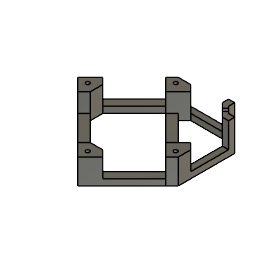
台2 v5 (Autodesk Fusion 360 design; units mm, degrees)
Autodesk Fusion 360 part; units mm, degrees
sketch "スケッチ1" plane through (0, 0, 0) normal (0, 0, 1) x (1, 0, 0)
  line L0 (0, 0) -> (-55, 0)
  line L1 (0, 0) -> (0, -5)
  line L2 (-10, -5) -> (-50, -5)
  line L3 (0, 0) -> (0, -55)
  line L4 (-5, -50) -> (-5, -10)
  line L5 (-5, -10) -> (-10, -5)
  line L6 (-5, -50) -> (-50, -5)
  line L7 (-5, -60) -> (-60, -5)
  line L8 (-60, -5) -> (-55, 0)
  line L9 (0, -55) -> (-5, -60)
  constraint coincident L0.start L1.start
  constraint horizontal L0
  constraint perpendicular L0 L1
  constraint perpendicular L1 L2
  constraint perpendicular L0 L3
  constraint perpendicular L2 L4
  constraint parallel L6 L7
  constraint perpendicular L6 L8
  constraint perpendicular L7 L9
extrude "押し出し1" add sketch "スケッチ1" along normal blind 5
sketch "スケッチ2" plane through (0, 0, 0) normal (0, 0, 1) x (1, 0, 0)
  line L0 (0, 0, 5) -> (-55, 0, 5)
  line L1 (-10, -5, 5) -> (-10, 0, 5)
  line L2 (-10, -5, 5) -> (-5, -10, 5)
  line L3 (0, -55, 5) -> (0, 0, 5)
  line L4 (-5, -10, 5) -> (0, -10, 5)
  line L5 (-60, -5, 5) -> (-5, -60, 5)
  line L6 (-5, -60, 5) -> (0, -55, 5)
  line L7 (-55, 0, 5) -> (-60, -5, 5)
  line L8 (-10, -55, 5) -> (-15, -50, 5)
  line L9 (-5, -10, 5) -> (-5, -50, 5)
  line L10 (0, -45, 5) -> (-5, -40, 5)
  line L11 (-15, -50, 5) -> (-5, -40, 5)
  line L12 (-50, -5, 5) -> (-10, -5, 5)
  line L13 (-50, -15, 5) -> (-40, -5, 5)
  line L14 (-45, 0, 5) -> (-40, -5, 5)
  line L15 (-55, -10, 5) -> (-50, -15, 5)
  point P0 (-10, -5)
  point P1 (-10, -5)
  point P2 (-5, -10)
  point P3 (-5, -50)
  point P4 (-50, -5)
  constraint coincident P0 P1
  constraint coincident P1 P0
extrude "押し出し2" add sketch "スケッチ2" along normal blind 50 contours L0 L1 L2 L3 L4 | L0 L5 L7 L13 L14 L15 | L3 L5 L6 L8 L10 L11 in plane through (0, 0, 5) normal (0, 0, 1)
sketch "スケッチ3" plane through (0, 0, 0) normal (0, 0, 1) x (1, 0, 0)
extrude "押し出し3" cut 2 faces at (-50, -5, 55) (-5, -50, 55) along direction (0, 0, -1) blind 30
sketch "スケッチ4" plane through (0, 0, 0) normal (0, 0, 1) x (1, 0, 0)
  line L0 (-60, -5) -> (-95, -40)
  line L1 (-95, -40) -> (-40, -95)
  line L2 (-40, -95) -> (-5, -60)
  line L3 (-5, -60) -> (-60, -5)
  line L4 (-55, -10) -> (-80, -35)
  line L5 (-80, -45) -> (-45, -80)
  line L6 (-35, -80) -> (-10, -55)
  line L7 (-35, -80) -> (-45, -80)
  line L8 (-80, -35) -> (-80, -45)
  point P0 (-5, -60)
  constraint perpendicular L0 L1
  constraint coincident P0 L2.end
  constraint coincident L3 L4.start
  constraint perpendicular L3 L4
  constraint perpendicular L4 L5
  constraint coincident L3 L6.end
  constraint perpendicular L3 L6
  constraint horizontal L7
  constraint perpendicular L7 L8
extrude "押し出し4" add sketch "スケッチ4" along normal blind 5 contours L0 L1 L2 L3 L4 L5 L6 L7 L8
sketch "スケッチ5" plane through (0, 0, 5) normal (0, 0, 1) x (-1, 0, 0)
  line L0 (55, 10) -> (60, 5)
  line L1 (60, 5) -> (95, 40)
  line L2 (95, 40) -> (40, 95)
  line L3 (40, 95) -> (5, 60)
  line L4 (10, 55) -> (35, 80)
  line L5 (35, 80) -> (45, 80)
  line L6 (45, 80) -> (80, 45)
  line L7 (80, 45) -> (80, 35)
  line L8 (80, 35) -> (55, 10)
  line L9 (80, 35) -> (85, 30)
  line L10 (80, 45) -> (85, 50)
  line L11 (45, 80) -> (50, 85)
  line L12 (35, 80) -> (30, 85)
  line L13 (5, 60) -> (10, 55)
  constraint coincident L7.end L8.start
  constraint coincident L1 L9.end
  constraint perpendicular L1 L9
  constraint coincident L6.end L7.start
  constraint coincident L2 L10.end
  constraint perpendicular L2 L10
  constraint coincident L5.end L6.start
  constraint coincident L2 L11.end
  constraint perpendicular L2 L11
  constraint coincident L4.end L5.start
  constraint coincident L3 L12.end
  constraint perpendicular L3 L12
extrude "押し出し5" add sketch "スケッチ5" along normal blind 20 contours L1 L2 L7 L9 L10 | L2 L3 L5 L11 L12
extrude "押し出し6" cut 4 faces at (-50, -5, 25) (-85, -40, 25) (-40, -85, 25) (-5, -50, 25) along direction (0, 0, -1) blind 5
extrude "押し出し7" add 2 faces at (-6.6667, -45, 5) (-45, -6.6667, 5) along direction (0, 0, -1) blind 5
sketch "スケッチ6" plane through (0, 0, 20) normal (0, 0, 1) x (-1, 0, 0)
  line L0 (45, 80) -> (50, 85)
  line L1 (50, 85) -> (40, 95)
  line L2 (40, 95) -> (30, 85)
  line L3 (30, 85) -> (35, 80)
  line L4 (35, 80) -> (45, 80)
  circle A0 centre (40, 87) radius 1.5
  circle A1 centre (5, 52) radius 1.5
  circle A2 centre (87, 40) radius 1.5
  circle A3 centre (52, 5) radius 1.5
extrude "押し出し8" cut sketch "スケッチ6" against normal blind 10 contours A0 | A1 | A2 | A3
extrude "押し出し9" cut 1 faces at (-5, -5, 55) along direction (0, 0, -1) blind 55
sketch "スケッチ7" plane through (0, 0, 0) normal (0, 0, 1) x (1, 0, 0)
  line L0 (-5, -10) -> (-10, -5)
  line L1 (-10, -5) -> (-15, -5)
  line L2 (-15, -5) -> (-5, -15)
  line L3 (-5, -15) -> (-5, -10)
  constraint horizontal L1
  constraint parallel L0 L2
  constraint perpendicular L1 L3
extrude "押し出し10" add sketch "スケッチ7" along normal blind 10
extrude "押し出し11" add 1 faces at (-5, -13.3333, 6.6667) along direction (1, 0, 0) blind 5
extrude "押し出し12" add 1 faces at (-11.6667, -5, 6.6667) along direction (0, 1, 0) blind 5
sketch "スケッチ8" plane through (-10, -10, 0) normal (-0.707107, -0.707107, 0) x (0.707107, -0.707107, 0)
  line L0 (-7.0711, 0) -> (7.0711, 0)
  line L1 (7.0711, 0) -> (7.0711, 5)
  line L2 (7.0711, 5) -> (7.0711, 10)
  line L3 (7.0711, 10) -> (-7.0711, 10)
  line L4 (-7.0711, 10) -> (-7.0711, 5)
  line L5 (-7.0711, 5) -> (-7.0711, 0)
extrude "押し出し13" add 1 faces at (-8.3333, -10, 10) along direction (0, 0, 1) blind 10
sketch "スケッチ9" plane through (-10, -10, 0) normal (-0.707107, -0.707107, 0) x (0.707107, -0.707107, 0)
  line L0 (-7.0711, 0) -> (7.0711, 0)
  line L1 (7.0711, 0) -> (7.0711, 5)
  line L2 (7.0711, 5) -> (7.0711, 20)
  line L3 (7.0711, 20) -> (-7.0711, 20)
  line L4 (-7.0711, 20) -> (-7.0711, 5)
  line L5 (-7.0711, 5) -> (-7.0711, 0)
  line L6 (0, 10) -> (0, 20)
  line L7 (1.5, 10) -> (1.5, 20)
  arc A0 (1.5, 20) -> (-1.5, 20) centre (0, 20) ccw
  line L8 (-1.5, 20) -> (-1.5, 10)
  arc A1 (-1.5, 10) -> (1.5, 10) centre (0, 10) ccw
  line L9 (0, 10) -> (0, 20) construction
  constraint midpoint L3 L6.end
  constraint perpendicular L3 L6
  constraint tangent L7 A0
  constraint tangent A0 L8
  constraint parallel L7 L8
  constraint tangent L8 A1
  constraint tangent L7 A1
  constraint coincident L6.end A0.centre
  constraint perpendicular L3 L9
  constraint coincident L6.start A1.centre
extrude "押し出し14" cut sketch "スケッチ9" against normal blind 4 contours L3 L7 L8 A1
extrude "押し出し15" add 2 faces at (-1.6667, -13.3333, 20) (-11.6667, -3.3333, 20) along direction (0, 0, 1) blind 5
